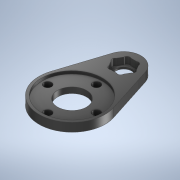
# Autodesk Inventor part: Slider_crank_horn
Saved by Autodesk Inventor 2022 (Build 260153000, 153)
## iProperties
Part Number: Slider_crank_horn
Material: アルミニウム 2014-T4
Document SubType Name: Modeling
Designer: Masato Kubotera
Density: 2.8 g/cm^3
Appearance: Smooth - Black
Description: A2017 T3
Mass: 3.09977 g
Surface Area: 14.8044 cm^2
Volume: 1.10706 cm^3
Author: Masato Kubotera
Revision Number: Rev.2 Specifications for RoboCup 2023: Anodized aluminum staining process added.
Autodesk Inventor part; units mm, degrees
ref_plane "YZ Plane" through (0, 0, 0) normal (1, 0, 0) x (0, 1, 0)
ref_plane "XZ Plane" through (0, 0, 0) normal (0, 1, 0) x (-1, 0, 0)
ref_plane "XY Plane" through (0, 0, 0) normal (0, 0, 1) x (1, 0, 0)
derived "Leg_joint_roll_basis.ipt"
sketch "スケッチ1" plane through (0, 0, 0) normal (0, 0, 1) x (1, 0, 0)
  line L0 (0, 47.5) -> (0, -12.4) construction
  line L1 (-12.5, 47.5) -> (12.5, 47.5) construction
  line L2 (-12.5, 42.45) -> (-5.9323, -0.8988) construction
  arc A0 (-5.9323, -0.8988) -> (5.9323, -0.8988) centre (0, 0) ccw construction
  line L3 (-5.55, 45.05) -> (-3.45, 45.05) construction
  line L4 (5.55, 45.05) -> (5.55, 42.45) construction
  line L5 (5.55, 42.45) -> (3.45, 42.45) construction
  line L6 (-5.55, 42.45) -> (-5.55, 45.05) construction
  line L7 (-5.55, 45.05) -> (5.55, 42.45) construction
  line L8 (5.55, 45.05) -> (-5.55, 42.45) construction
  line L9 (-5.5, 45) -> (5.5, 45) construction
  line L10 (5.5, 45) -> (5.5, 42.5) construction
  line L11 (5.5, 42.5) -> (-5.5, 42.5) construction
  line L12 (-5.5, 42.5) -> (-5.5, 45) construction
  line L13 (-5.5, 45) -> (5.5, 42.5) construction
  line L14 (5.5, 45) -> (-5.5, 42.5) construction
  line L15 (-5.55, 43.75) -> (5.55, 43.75) construction
  arc A1 (-3.45, 45.05) -> (-5.55, 45.05) centre (-4.5, 45.05) ccw construction
  arc A2 (-5.55, 42.45) -> (-3.45, 42.45) centre (-4.5, 42.45) ccw construction
  line L16 (12.5, 42.45) -> (5.9323, -0.8988) construction
  arc A3 (5.55, 45.05) -> (3.45, 45.05) centre (4.5, 45.05) ccw construction
  arc A4 (3.45, 42.45) -> (5.55, 42.45) centre (4.5, 42.45) ccw construction
  line L17 (-3.45, 45.05) -> (3.45, 45.05) construction
  line L18 (-3.45, 42.45) -> (-5.55, 42.45) construction
  line L19 (3.45, 42.45) -> (-3.45, 42.45) construction
  line L20 (3.45, 45.05) -> (5.55, 45.05) construction
  circle A5 centre (0, 0) radius 4.05 construction
  line L21 (-13.5, 17) -> (13.5, 17) construction
  line L22 (13.5, 17) -> (13.5, -10) construction
  line L23 (13.5, -10) -> (-13.5, -10) construction
  line L24 (-13.5, -10) -> (-13.5, 17) construction
  line L25 (-13.5, 17) -> (13.5, -10) construction
  line L26 (13.5, 17) -> (-13.5, -10) construction
  arc A6 (-13.5, 18.35) -> (-13.5, 15.65) centre (-13.5, 17) ccw construction
  circle A7 centre (-13.5, -10) radius 1.35 construction
  line L27 (-24.825, 12.5) -> (-24.825, -5.5) construction
  circle A8 centre (-13.5, -10) radius 2.4 construction
  line L28 (-24.825, -5.5) -> (-14.2116, -12.4) construction
  line L29 (-21.75, 7.5) -> (-19.75, 7.5) construction
  line L30 (-19.75, 7.5) -> (-19.75, -0.5) construction
  line L31 (-19.75, -0.5) -> (-21.75, -0.5) construction
  line L32 (-21.75, -0.5) -> (-21.75, 7.5) construction
  line L33 (-21.75, 7.5) -> (-19.75, -0.5) construction
  line L34 (-19.75, 7.5) -> (-21.75, -0.5) construction
  line L35 (-21.775, 7.525) -> (-19.725, 7.525) construction
  line L36 (-19.725, 7.525) -> (-19.725, 5.425) construction
  line L37 (-19.725, -0.525) -> (-21.775, -0.525) construction
  line L38 (-21.775, -0.525) -> (-21.775, 1.575) construction
  line L39 (-21.775, 7.525) -> (-19.725, -0.525) construction
  line L40 (-19.725, 7.525) -> (-21.775, -0.525) construction
  arc A9 (-21.775, 7.525) -> (-21.775, 5.425) centre (-21.775, 6.475) ccw construction
  line L41 (-20.75, 7.525) -> (-20.75, -0.525) construction
  line L42 (-21.76, 3.5) -> (-19.74, 3.5) construction
  arc A10 (-19.725, 5.425) -> (-19.725, 7.525) centre (-19.725, 6.475) ccw construction
  arc A11 (-21.775, 1.575) -> (-21.775, -0.525) centre (-21.775, 0.525) ccw construction
  arc A12 (-19.725, -0.525) -> (-19.725, 1.575) centre (-19.725, 0.525) ccw construction
  line L43 (-24.825, 12.5) -> (-14.2116, 19.4) construction
  line L44 (-13.5, 18.35) -> (-13, 18.35) construction
  line L45 (-13.5, 15.65) -> (-13, 15.65) construction
  arc A13 (-13, 15.65) -> (-13, 18.35) centre (-13, 17) ccw construction
  line L46 (-21.775, 5.425) -> (-21.775, 7.525) construction
  line L47 (-21.775, 1.575) -> (-21.775, 5.425) construction
  line L48 (-19.725, 1.575) -> (-19.725, -0.525) construction
  line L49 (-19.725, 5.425) -> (-19.725, 1.575) construction
  line L50 (19.725, 5.425) -> (19.725, 1.575) construction
  line L51 (21.775, 1.575) -> (21.775, 5.425) construction
  arc A14 (21.775, 5.425) -> (21.775, 7.525) centre (21.775, 6.475) ccw construction
  line L52 (21.775, 7.525) -> (19.725, 7.525) construction
  arc A15 (19.725, 7.525) -> (19.725, 5.425) centre (19.725, 6.475) ccw construction
  arc A16 (21.775, -0.525) -> (21.775, 1.575) centre (21.775, 0.525) ccw construction
  line L53 (19.725, -0.525) -> (21.775, -0.525) construction
  arc A17 (19.725, 1.575) -> (19.725, -0.525) centre (19.725, 0.525) ccw construction
  line L54 (24.825, 12.5) -> (24.825, -5.5) construction
  line L55 (24.825, 12.5) -> (14.2116, 19.4) construction
  arc A18 (13, 18.35) -> (13, 15.65) centre (13, 17) ccw construction
  line L56 (13.5, 18.35) -> (13, 18.35) construction
  arc A19 (13.5, 15.65) -> (13.5, 18.35) centre (13.5, 17) ccw construction
  line L57 (24.825, -5.5) -> (14.2116, -12.4) construction
  circle A20 centre (13.5, -10) radius 1.35 construction
  line L58 (13.5, 15.65) -> (13, 15.65) construction
  line L59 (-14.2116, -12.4) -> (14.2116, -12.4) construction
  line L60 (-14.2116, 19.4) -> (-11.0486, 19.4) construction
  circle A21 centre (0, 18) radius 5.05
  circle A22 centre (-13.5, 17) radius 2.4 construction
  arc A23 (-11.0486, 19.4) -> (11.0486, 19.4) centre (0, 18) ccw construction
  line L61 (11.0486, 19.4) -> (14.2116, 19.4) construction
  circle A24 centre (0, 26.5) radius 1.35
  circle A25 centre (-8.5, 18) radius 1.35
  circle A26 centre (0, 9.5) radius 1.35
  circle A27 centre (8.5, 18) radius 1.35
  arc A28 (5.713, 37.8333) -> (-5.713, 37.8333) centre (0, 36) ccw
  circle A29 centre (0, 36) radius 2.75
  circle A30 centre (0, 0) radius 2.75 construction
  circle A31 centre (0, 0) radius 2.1 construction
  line L62 (0, -4.053) -> (-0.9093, -3.528) construction
  line L63 (-3.51, -2.0265) -> (-3.51, -0.9765) construction
  line L64 (-3.51, 2.0265) -> (-2.6007, 2.5515) construction
  line L65 (0, 4.053) -> (3.51, 2.0265) construction
  line L66 (3.51, 2.0265) -> (3.51, 0.9765) construction
  line L67 (3.51, -2.0265) -> (2.6007, -2.5515) construction
  arc A32 (0.9093, 3.528) -> (-0.9093, 3.528) centre (0, 3.003) ccw construction
  arc A33 (-2.6007, 2.5515) -> (-3.51, 0.9765) centre (-2.6007, 1.5015) ccw construction
  arc A34 (-3.51, -0.9765) -> (-2.6007, -2.5515) centre (-2.6007, -1.5015) ccw construction
  arc A35 (-0.9093, -3.528) -> (0.9093, -3.528) centre (0, -3.003) ccw construction
  arc A36 (2.6007, -2.5515) -> (3.51, -0.9765) centre (2.6007, -1.5015) ccw construction
  arc A37 (3.51, 0.9765) -> (2.6007, 2.5515) centre (2.6007, 1.5015) ccw construction
  line L68 (-0.9093, 3.528) -> (0, 4.053) construction
  line L69 (-2.6007, 2.5515) -> (-0.9093, 3.528) construction
  line L70 (-3.51, 0.9765) -> (-3.51, 2.0265) construction
  line L71 (-3.51, -0.9765) -> (-3.51, 0.9765) construction
  line L72 (-2.6007, -2.5515) -> (-3.51, -2.0265) construction
  line L73 (-0.9093, -3.528) -> (-2.6007, -2.5515) construction
  line L74 (0.9093, -3.528) -> (0, -4.053) construction
  line L75 (2.6007, -2.5515) -> (0.9093, -3.528) construction
  line L76 (3.51, -0.9765) -> (3.51, -2.0265) construction
  line L77 (3.51, 0.9765) -> (3.51, -0.9765) construction
  circle A38 centre (0, 0) radius 3 construction
  circle A39 centre (-9.5, 45) radius 1.6 construction
  circle A40 centre (9.5, 45) radius 1.6 construction
  line L78 (-12.5, 42.45) -> (-12.5, 47.5) construction
  line L79 (12.5, 47.5) -> (12.5, 42.45) construction
  arc A41 (-8.4171, 15.5014) -> (-9.1609, 20.4111) centre (-8.5, 18) ccw construction
  arc A42 (9.1609, 20.4111) -> (8.4171, 15.5014) centre (8.5, 18) ccw construction
  circle A43 centre (0, 9.5) radius 2.5 construction
  circle A44 centre (0, 18) radius 10.55
  circle A45 centre (0, 18) radius 11.5
  line L80 (-10.95, 21.5139) -> (-5.713, 37.8333)
  line L81 (5.713, 37.8333) -> (10.95, 21.5139)
  line L82 (2.0265, 32.49) -> (0.9765, 32.49) construction
  line L83 (-2.0265, 32.49) -> (-2.5515, 33.3993) construction
  line L84 (-4.053, 36) -> (-3.528, 36.9093) construction
  line L85 (-2.0265, 39.51) -> (-0.9765, 39.51) construction
  line L86 (2.0265, 39.51) -> (2.5515, 38.6007) construction
  line L87 (4.053, 36) -> (3.528, 35.0907) construction
  arc A46 (-0.9765, 39.51) -> (-2.5515, 38.6007) centre (-1.5015, 38.6007) ccw
  arc A47 (-3.528, 36.9093) -> (-3.528, 35.0907) centre (-3.003, 36) ccw
  arc A48 (-2.5515, 33.3993) -> (-0.9765, 32.49) centre (-1.5015, 33.3993) ccw
  arc A49 (0.9765, 32.49) -> (2.5515, 33.3993) centre (1.5015, 33.3993) ccw
  arc A50 (3.528, 35.0907) -> (3.528, 36.9093) centre (3.003, 36) ccw
  arc A51 (2.5515, 38.6007) -> (0.9765, 39.51) centre (1.5015, 38.6007) ccw
  line L88 (-2.5515, 38.6007) -> (-2.0265, 39.51) construction
  line L89 (-3.528, 36.9093) -> (-2.5515, 38.6007)
  line L90 (-3.528, 35.0907) -> (-4.053, 36) construction
  line L91 (-2.5515, 33.3993) -> (-3.528, 35.0907)
  line L92 (-0.9765, 32.49) -> (-2.0265, 32.49) construction
  line L93 (0.9765, 32.49) -> (-0.9765, 32.49)
  line L94 (2.5515, 33.3993) -> (2.0265, 32.49) construction
  line L95 (3.528, 35.0907) -> (2.5515, 33.3993)
  line L96 (3.528, 36.9093) -> (4.053, 36) construction
  line L97 (2.5515, 38.6007) -> (3.528, 36.9093)
  line L98 (-0.9765, 39.51) -> (0.9765, 39.51)
  line L99 (0.9765, 39.51) -> (2.0265, 39.51) construction
  circle A52 centre (0, 0) radius 6 construction
  point P0 (0, 43.75)
  point P1 (0, 3.5)
  point P2 (-20.75, 3.5)
  point P3 (-24.825, 3.5)
  point P4 (-13.5, 3.5)
extrude "押し出し1" add sketch "スケッチ1" along normal blind 3 contours L81 A45 L80 A28 | A45
extrude "押し出し2" add sketch "スケッチ1" along normal blind 2 contours A44
extrude "押し出し3" add sketch "スケッチ1" along normal blind 0.6 contours L98 A51 L97 A50 L95 A49 L93 A48 L91 A47 L89 A46
